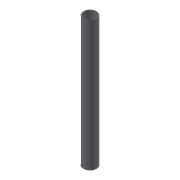
# Autodesk Inventor part: 50mm Tubing
Saved by Autodesk Inventor 2015 (Build 190159000, 159)
## iProperties
Created: 2020-04-22
Part Number: 50mm Tubing
Material: Aluminum 6061-AHC
Document SubType Name: Modeling
Designer: Ghassan Yusuf
Density: 2.7 g/cm^3
Appearance: Aluminum - Dark
Author: Ghassan Yusuf
Autodesk Inventor part; units mm, degrees
ref_plane "YZ Plane" through (0, 0, 0) normal (1, 0, 0) x (0, 1, 0)
ref_plane "XZ Plane" through (0, 0, 0) normal (0, 1, 0) x (-1, 0, 0)
ref_plane "XY Plane" through (0, 0, 0) normal (0, 0, 1) x (1, 0, 0)
sketch "Sketch1" plane through (0, 0, 0) normal (0, 0, 1) x (1, 0, 0)
  circle A0 centre (0, 0) radius 25
  circle A1 centre (0, 0) radius 22.5
  dimension "d0" = 50
  dimension "d1" = 2.5
  constraints: 2 centre point, 1 coincident
  measures "d0" diameter of A0
  measures "d1" radial gap between concentric circles of A0 A1
extrude "Extrusion1" add sketch "Sketch1" along normal mid plane 500
body "Solid1"
